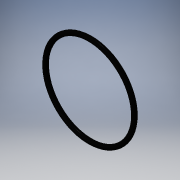
# Autodesk Inventor part: ORING
Saved by Autodesk Inventor 2016 (Build 200138000, 138)
## iProperties
Created: 2016-10-13
Part Number: ORING
Material: Generic
Document SubType Name: Modeling
Designer: brandn
Density: 1 g/cm^3
Appearance: Default
Author: brandn
Autodesk Inventor part; units mm, degrees
ref_plane "YZ Plane" through (0, 0, 0) normal (1, 0, 0) x (0, 1, 0)
ref_plane "XZ Plane" through (0, 0, 0) normal (0, 1, 0) x (-1, 0, 0)
ref_plane "XY Plane" through (0, 0, 0) normal (0, 0, 1) x (1, 0, 0)
sketch "Sketch1" plane through (0, 0, 0) normal (1, 0, 0) x (0, 1, 0)
  circle A0 centre (33.3121, 0) radius 1.7653
  line L0 (0, 0) -> (0, -13.7103)
  dimension "d0" = 3.5306
  dimension "d1" = 63.0936
  constraints: 2 end point, 1 centre point, 1 vertical
  measures "d0" diameter of A0
revolve "Revolution1" add sketch "Sketch1" angle 360 about axis through (0, 0, 0) along (0, 0, -1)
body "Solid1"
